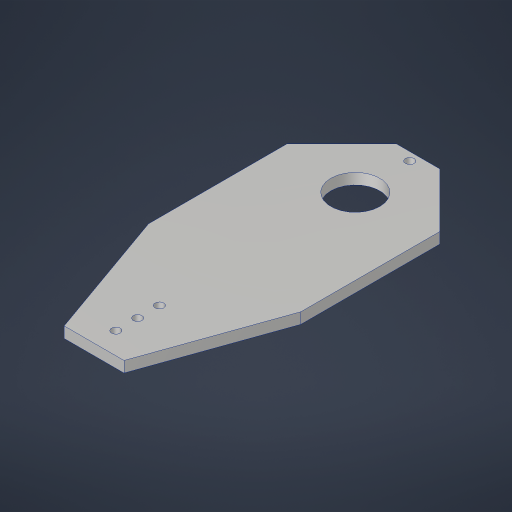
# Autodesk Inventor part: CL4-002
Saved by Autodesk Inventor 2023.4 (Build 274418000, 418)
## iProperties
Created: 2025-02-04
Part Number: CL4-002
Material: Aluminum 6061
Document SubType Name: Modeling
Designer: brand
Density: 2.7 g/cm^3
Appearance: Aluminum - Flat
Author: brand
Autodesk Inventor part; units mm, degrees
ref_plane "YZ Plane" through (0, 0, 0) normal (1, 0, 0) x (0, 1, 0)
ref_plane "XZ Plane" through (0, 0, 0) normal (0, 1, 0) x (-1, 0, 0)
ref_plane "XY Plane" through (0, 0, 0) normal (0, 0, 1) x (1, 0, 0)
sketch "Sketch1" plane through (0, 0, 0) normal (0, 1, 0) x (-1, 0, 0)
  line L0 (44.45, 0) -> (-44.45, 0)
  line L1 (-44.45, 0) -> (-44.45, -188.9125)
  line L2 (-44.45, -188.9125) -> (44.45, -188.9125)
  line L3 (44.45, -188.9125) -> (44.45, 0)
  line L4 (12.7, -50.8) -> (-12.7, -50.8) construction
  line L5 (-12.7, -50.8) -> (-12.7, 0) construction
  line L6 (-12.7, 0) -> (12.7, 0) construction
  line L7 (12.7, 0) -> (12.7, -50.8) construction
  circle A0 centre (0, -152.4) radius 14.2875
  circle A1 centre (0, -184.15) radius 4.7625 construction
  point P0 (0, 0)
  point P1 (0, 0)
  dimension "d0" = 50.8
  dimension "d1" = 25.4
  dimension "d2" = 88.9
  dimension "d4" = 28.575
  dimension "d5" = 9.525
  dimension "d6" = 31.75
  dimension "d7" = 152.4
  constraints: 16 end point, 4 parallel, 2 centre point, 2 horizontal, 2 midpoint, 2 perpendicular, 2 vertical alignment, 1 coincident, 1 tangent
  measures "d0" distance of L6.end L4.start
  measures "d1" distance of L5.end L6.end
  measures "d2" distance of L0.start L0.end
  measures "d4" diameter of A0
  measures "d5" diameter of A1
  measures "d6" distance of A0.centre A1.centre
  measures "d7" distance of point (0, 0) A0.centre
extrude "Extrusion1" add sketch "Sketch1" against normal blind 6.35
hole "Hole1" at (0, 0, -184.15) direction (0, -1, 0) diameter 5.1054 end through all clearance for "Flat Head Machine Screw (82)" size "#10" standard "Ansi Unified Screw Threads"
sketch "Sketch2" plane through (0, 0, 0) normal (0, 1, 0) x (1, 0, 0)
  circle A0 centre (0, 184.15) radius 2.5527 construction
  circle A1 centre (0, 152.4) radius 14.2875 construction
  line L0 (-44.45, 188.9125) -> (44.45, 188.9125) construction
  line L1 (44.45, 188.9125) -> (44.45, 0) construction
  line L2 (44.45, 0) -> (-44.45, 0) construction
  line L3 (-44.45, 0) -> (-44.45, 188.9125) construction
  line L4 (-44.45, 188.9125) -> (-44.45, 0) construction
  line L5 (-44.45, 157.1625) -> (-12.7, 188.9125)
  line L6 (44.45, 188.9125) -> (-44.45, 188.9125) construction
  line L7 (-12.7, 188.9125) -> (-44.45, 188.9125)
  line L8 (-44.45, 157.1625) -> (-44.45, 188.9125)
  line L9 (44.45, 188.9125) -> (12.7, 188.9125)
  line L10 (12.7, 188.9125) -> (44.45, 157.1625)
  line L11 (44.45, 157.1625) -> (44.45, 188.9125)
  line L12 (44.45, 0) -> (44.45, 188.9125) construction
  line L13 (-12.7, 188.9125) -> (12.7, 188.9125) construction
  line L14 (-44.45, 0) -> (-17.4625, 0)
  line L15 (-17.4625, 0) -> (-44.45, 76.2)
  line L16 (-44.45, 76.2) -> (-44.45, 0)
  line L17 (17.4625, 0) -> (44.45, 0)
  line L18 (44.45, 0) -> (44.45, 76.2)
  line L19 (44.45, 76.2) -> (17.4625, 0)
  line L20 (-44.45, 0) -> (44.45, 0) construction
  line L21 (-12.7, 0) -> (12.7, 0) construction
  line L22 (12.7, 0) -> (12.7, 50.8) construction
  line L23 (12.7, 50.8) -> (-12.7, 50.8) construction
  line L24 (-12.7, 50.8) -> (-12.7, 0) construction
  line L25 (17.4625, 0) -> (-17.4625, 0) construction
  point P0 (0, 0)
  point P1 (0, 188.9125)
  point P2 (0, 50.8)
  point P3 (0, 0)
  point P4 (0, 0)
  point P5 (0, 0)
  point P6 (0, 0)
  dimension "d18" = 25.4
  dimension "d19" = 31.75
  dimension "d20" = 31.75
  dimension "d21" = 25.4
  dimension "d22" = 50.8
  dimension "d23" = 34.925
  dimension "d24" = 76.2
  constraints: 36 end point, 11 point on line, 6 midpoint, 5 perpendicular, 4 horizontal, 3 collinear, 3 vertical alignment, 2 horizontal alignment, 2 parallel, 1 coincident
  measures "d18" distance of L9.end L5.end
  measures "d19" distance of L0.start L5.end
  measures "d20" distance of L5.start L0.start
  measures "d21" distance of L22.end L23.end
  measures "d22" distance of L23.end L21.start
  measures "d23" distance of L17.start L14.end
  measures "d24" distance of L14.start L15.end
extrude "Extrusion2" cut sketch "Sketch2" against normal through all
sketch "Sketch3" plane through (0, 0, 0) normal (0, 1, 0) x (1, 0, 0)
  line L0 (-17.4625, 0) -> (17.4625, 0) construction
  line L1 (0, 12.7) -> (0, 38.1) construction
  point P0 (0, 0)
  point P1 (0, 25.4)
  point P2 (0, 0)
  point P3 (0, 0)
  point P4 (0, 25.4)
  dimension "d27" = 12.7
  dimension "d28" = 25.4
  constraints: 3 midpoint, 3 vertical alignment, 2 end point, 1 coincident, 1 vertical
  measures "d27" distance of point (0, 0) L1.start
  measures "d28" distance of L1.start L1.end
hole "Hole2" at (0, 0, -12.7) at (0, 0, -25.4) at (0, 0, -38.1) direction (0, -1, 0) diameter 5.1054 end through all clearance for "Flat Head Machine Screw (82)" size "#10" standard "Ansi Unified Screw Threads"
equation "\"d20\" = d19"
body "Solid1"
